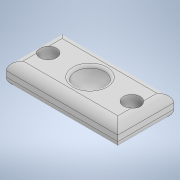
# Autodesk Inventor part: TestBearingPad
Saved by Autodesk Inventor 2022 (Build 260153000, 153)
## iProperties
Created: 2022-03-11
Part Number: TestBearingPad
Material: Generic
Document SubType Name: Modeling
Designer: Jorian Brusind
Density: 1 g/cm^3
Appearance: Default
Author: Jorian Brusind
Autodesk Inventor part; units mm, degrees
ref_plane "YZ Plane" through (0, 0, 0) normal (1, 0, 0) x (0, 1, 0)
ref_plane "XZ Plane" through (0, 0, 0) normal (0, 1, 0) x (-1, 0, 0)
ref_plane "XY Plane" through (0, 0, 0) normal (0, 0, 1) x (1, 0, 0)
sketch "Sketch1" plane through (0, 0, 0) normal (0, 1, 0) x (-1, 0, 0)
  line L0 (-20, -10) -> (20, -10)
  line L1 (20, -10) -> (20, 10)
  line L2 (20, 10) -> (-20, 10)
  line L3 (-20, 10) -> (-20, -10)
  line L4 (-20, -10) -> (20, 10) construction
  line L5 (20, -10) -> (-20, 10) construction
  point P0 (0, 0)
  dimension "d0" = 40
  dimension "d1" = 20
  constraints: 12 end point, 2 midpoint, 2 parallel, 1 horizontal, 1 perpendicular
  measures "d0" distance of L2.end L1.end
  measures "d1" distance of L1.end L0.end
extrude "Extrusion1" add sketch "Sketch1" along normal blind 8
ref_plane "Work Plane1" through (-20, 0, 0) normal (0, 0, 1) x (1, 0, 0)
sketch "Sketch3" plane through (-20, 0, 0) normal (0, 0, 1) x (1, 0, 0)
  line L0 (0, 8) -> (40, 8) projected
  line L1 (40, 8) -> (30, 8)
  circle A0 centre (20, 8) radius 5.25
  line L2 (0, 0) -> (40, 0) projected
  line L3 (20, 8) -> (20, 10)
  line L4 (20, 10) -> (15.1459, 10)
  line L5 (20, 10) -> (24.8541, 10)
  line L6 (20, 8) -> (20, 2.75)
  point P0 (20, 0)
  dimension "d12" = 10
  dimension "d13" = 10.5
  dimension "d14" = 8
  dimension "d15" = 20
  dimension "d16" = 2
  dimension "d17" = 5.25
  constraints: 10 end point, 2 point on circle, 2 point on line, 2 vertical, 1 centre point, 1 perpendicular
  measures "d12" distance of L0.end L1.end
  measures "d13" diameter of A0
  measures "d14" distance from line of L2 L3.start
  measures "d15" distance of L0.end L3.start
  measures "d16" distance of L3.start L3.end
  measures "d17" distance of L3.start L6.end
revolve "Revolution3" cut sketch "Sketch3" angle 360 about axis through (0, 8, 0) along (0, 1, 0) picked at (23.4561, 7.6106) contours L3 L5 A0 L0 | L0 A0 L6
fillet "Fillet2" radius 1 1 edges at (-5.25, 8, 0)
pattern_of_one "Rectangular Pattern2"
sketch "Sketch4" plane through (0, 8, 0) normal (0, 1, 0) x (1, 0, 0)
  line L0 (-20, 10) -> (-20, -10) projected
  line L1 (-20, 0) -> (-15, 0)
  line L2 (20, -10) -> (20, 10) projected
  line L3 (20, 0) -> (15, 0)
  circle A0 centre (-15, 0) radius 3
  circle A1 centre (15, 0) radius 3
  point P0 (0, 0)
  dimension "d33" = 5
  dimension "d34" = 5
  dimension "d35" = 6
  dimension "d36" = 6
  constraints: 4 end point, 2 centre point, 2 coincident, 2 horizontal, 2 midpoint
  measures "d33" distance of L1.start L1.end
  measures "d34" distance of L3.start L3.end
  measures "d35" diameter of A0
  measures "d36" diameter of A1
extrude "Extrusion2" cut sketch "Sketch4" against normal blind 10
fillet "Fillet3" radius 3 4 edges at (0, 8, 10) (0, 8, -10) (-20, 8, 0) (20, 8, 0)
fillet "Fillet4" radius 3 4 edges at (0, 0, 10) (-20, 0, 0) (20, 0, 0) (0, 0, -10)
body "Solid1"
